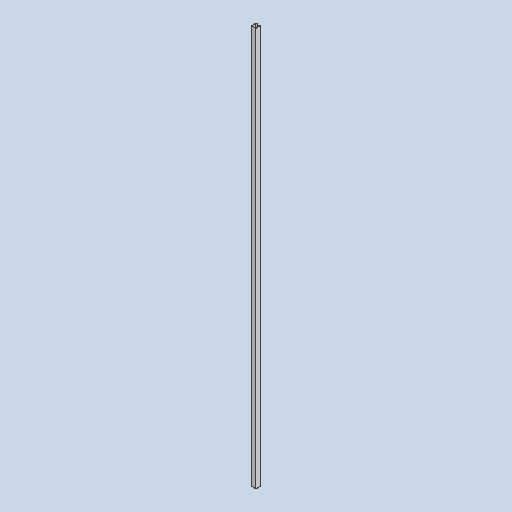
# Autodesk Inventor part: guiaPorta
Saved by Autodesk Inventor 2023 (Build 270158000, 158)
## iProperties
Created: 2022-08-29
Part Number: guiaPorta
Material: Generic
Document SubType Name: Modeling
Designer: cvss2
Density: 1 g/cm^3
Appearance: Default
Author: cvss2
Autodesk Inventor part; units mm, degrees
ref_plane "YZ Plane" through (0, 0, 0) normal (1, 0, 0) x (0, 1, 0)
ref_plane "XZ Plane" through (0, 0, 0) normal (0, 1, 0) x (-1, 0, 0)
ref_plane "XY Plane" through (0, 0, 0) normal (0, 0, 1) x (1, 0, 0)
sketch "Sketch1" plane through (0, 0, 0) normal (0, 1, 0) x (-1, 0, 0)
  line L0 (0, 0) -> (-30, 0)
  line L1 (-30, 0) -> (-30, 30)
  line L2 (-30, 30) -> (0, 30)
  line L3 (0, 30) -> (0, 0)
  line L4 (-2, 28) -> (-28, 28)
  line L5 (-28, 28) -> (-28, 2)
  line L6 (-28, 2) -> (-2, 2)
  line L7 (-2, 2) -> (-2, 28)
  line L8 (-10, 0) -> (-20, 0)
  line L9 (-20, 0) -> (-20, 30)
  line L10 (-20, 30) -> (-10, 30)
  line L11 (-10, 30) -> (-10, 0)
  line L12 (-10, 0) -> (-20, 30) construction
  line L13 (-20, 0) -> (-10, 30) construction
  point P0 (-15, 15)
  point P1 (-20, 2)
  point P2 (-10, 2)
  dimension "d0" = 30
  dimension "d1" = 30
  dimension "d2" = 2
  dimension "d3" = 10
  dimension "d4" = 30
  dimension "d5" = 15
  constraints: 28 end point, 6 parallel, 3 perpendicular, 2 horizontal, 2 midpoint, 3 other
  measures "d0" distance of L1.end L2.end
  measures "d1" distance of L0.end L1.end
  measures "d2" distance between parallel lines of L2 L4
  measures "d3" distance of L9.end L10.end
  measures "d4" distance of L8.end L9.end
  measures "d5" distance from line of L3 point (-15, 15)
extrude "Extrusion1" add sketch "Sketch1" along normal blind 2560 contours L0 L11 L6 L7 L4 L2 L3 | L0 L1 L2 L9 L4 L5 L6 | L11 L4 L9 L2
sketch "Sketch2" plane through (20, 0, 0) normal (0, 0, -1) x (-1, 0, 0)
  line L0 (-10, 0) -> (0, 0) projected
  line L1 (0, 0) -> (0, 2560) projected
  line L2 (-10, 2560) -> (0, 2560) projected
  line L3 (-10, 0) -> (-10, 2560) projected
  line L4 (10, 0) -> (20, 0) projected
  line L5 (20, 0) -> (20, 2560) projected
  line L6 (10, 2560) -> (20, 2560) projected
  line L7 (10, 0) -> (10, 2560) projected
  line L8 (-8, 2560) -> (18, 2560) construction
  line L9 (5, 2560) -> (5, 2050) construction
  circle A0 centre (5, 2050) radius 7.5
  line L10 (-8, 0) -> (18, 0) construction
  line L11 (5, 0) -> (5, 510) construction
  circle A1 centre (5, 510) radius 7.5
  point P0 (10, 2055.5902)
  point P1 (10, 2044.4098)
  point P2 (0, 2055.5902)
  point P3 (0, 2044.4098)
  point P4 (10, 515.5902)
  point P5 (10, 504.4098)
  point P6 (0, 515.5902)
  point P7 (0, 504.4098)
  dimension "d8" = 510
  dimension "d9" = 15
  dimension "d10" = 510
  dimension "d11" = 15
  constraints: 4 end point, 2 centre point, 2 coincident, 2 midpoint, 2 vertical
  measures "d8" distance of L9.start L9.end
  measures "d9" diameter of A0
  measures "d10" distance of L11.start L11.end
  measures "d11" diameter of A1
extrude "Extrusion2" cut sketch "Sketch2" against normal up to surface (2 mm away) contours A1 L1 | L7 A1 | L1 A0 | A0 L7
equation "\"d4\" = d1"
equation "\"d5\" = 0.5 * d1"
equation "\"d10\" = d8"
body "Solid1"
